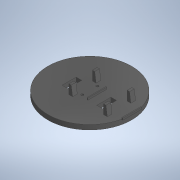
# Autodesk Inventor part: Swivel Top Drafting
Saved by Autodesk Inventor 2020.5 (Build 245400000, 400)
## iProperties
Part Number: Swivel Top Drafting
Material: Generic
Document SubType Name: Modeling
Designer: Wes
Appearance: Default
Author: Wes
Autodesk Inventor part; units mm, degrees
ref_plane "YZ Plane" through (0, 0, 0) normal (1, 0, 0) x (0, 1, 0)
ref_plane "XZ Plane" through (0, 0, 0) normal (0, 1, 0) x (-1, 0, 0)
ref_plane "XY Plane" through (0, 0, 0) normal (0, 0, 1) x (1, 0, 0)
sketch "Sketch1" plane through (0, 0, 0) normal (0, 0, 1) x (1, 0, 0)
  line L0 (0, 0) -> (0, 120) construction
  line L1 (-22.9924, 0) -> (-22.9924, 62) construction
  circle A0 centre (0, 31) radius 89
  line L2 (-20, 119) -> (20, 119)
  line L3 (20, 119) -> (20, 121)
  line L4 (20, 121) -> (-20, 121)
  line L5 (-20, 121) -> (-20, 119)
  line L6 (-20, 119) -> (20, 121) construction
  line L7 (20, 119) -> (-20, 121) construction
  line L8 (3.5475, 119) -> (3.5475, 78) construction
  line L9 (3.5475, 78) -> (3.5475, 66) construction
  line L10 (-20, 72) -> (-10, 72) construction
  line L11 (20, 72) -> (29, 72) construction
  line L12 (20, 66) -> (-10, 66)
  line L13 (-10, 66) -> (-10, 78)
  line L14 (-10, 78) -> (20, 78)
  line L15 (20, 78) -> (20, 66)
  line L16 (-20, 45.1356) -> (20, 45.1356)
  line L17 (20, 47.1356) -> (-20, 47.1356)
  line L18 (20, -7.8644) -> (-10, -7.8644)
  line L19 (-10, -7.8644) -> (-10, 4.1356)
  line L20 (-10, 4.1356) -> (20, 4.1356)
  line L21 (20, 4.1356) -> (20, -7.8644)
  line L22 (-20, 45.1356) -> (-20, 47.1356)
  line L23 (20, 45.1356) -> (20, 47.1356)
  line L24 (0, 31) -> (-16, 31) construction
  line L25 (0, 31) -> (16, 31) construction
  circle A1 centre (16, 31) radius 1.15
  circle A2 centre (-16, 31) radius 1.15
  point P0 (13.3041, 119)
  point P1 (-13.3041, 119)
  dimension "d0" = 120
  dimension "d1" = 62
  dimension "d2" = 40
  dimension "d3" = 2
  dimension "d4" = 41
  dimension "d5" = 12
  dimension "d6" = 10
  dimension "d7" = 9
  dimension "d8" = 30
  dimension "d9" = 12
  dimension "d10" = 40
  dimension "d11" = 2
  dimension "d12" = 30
  dimension "d13" = 12
  dimension "d18" = 16
  dimension "d19" = 16
  dimension "d20" = 2.3
  dimension "d21" = 2.3
  constraints: 52 end point, 8 horizontal, 7 parallel, 5 vertical, 4 perpendicular, 2 centre point, 2 coincident, 2 midpoint, 2 point on line, 3 other
  measures "d0" distance of L0.start L0.end
  measures "d1" distance of L1.start L1.end
  measures "d2" distance of L4.end L3.end
  measures "d3" distance of L3.end L2.end
  measures "d4" distance of L8.start L8.end
  measures "d5" distance of L8.end L9.end
  measures "d6" distance of L10.start L10.end
  measures "d7" distance of L11.start L11.end
  measures "d8" distance of L13.end L14.end
  measures "d9" distance of L12.end L13.end
  measures "d10" distance of L17.end L17.start
  measures "d11" distance of L17.start L16.end
  measures "d12" distance of L19.end L20.end
  measures "d13" distance of L19.start L19.end
  measures "d18" distance of L24.start L24.end
  measures "d19" distance of L24.start L25.end
  measures "d20" diameter of A1
  measures "d21" diameter of A2
extrude "Extrusion1" add sketch "Sketch1" along normal mid plane 10 contours A0 L2 | L2 A0 | L22 L17 L23 L16
sketch "Sketch2" plane through (0, 0, 5) normal (0, 0, 1) x (1, 0, 0)
  line L0 (20, 121) -> (-20, 121) projected
  line L1 (-20, 121) -> (-20, 119) projected
  line L2 (-20, 119) -> (20, 119) projected
  line L3 (20, 119) -> (20, 121) projected
  line L4 (20, 45.1356) -> (-20, 45.1356) projected
  line L5 (-20, 45.1356) -> (-20, 47.1356) projected
  line L6 (-20, 47.1356) -> (20, 47.1356) projected
  line L7 (20, 47.1356) -> (20, 45.1356) projected
  point P0 (0, 0)
extrude "Extrusion2" add sketch "Sketch2" along normal blind 4
sketch "Sketch3" plane through (0, 0, 5) normal (0, 0, 1) x (1, 0, 0)
  circle A0 centre (-16, 31) radius 2.65
  circle A1 centre (16, 31) radius 2.65
  point P0 (0, 0)
  dimension "d22" = 5.3
  dimension "d23" = 5.3
  constraints: 2 centre point, 2 coincident
  measures "d22" diameter of A0
  measures "d23" diameter of A1
extrude "Extrusion3" cut sketch "Sketch3" against normal blind 2.2
sketch "Sketch4" plane through (0, 31, -5) normal (0, 0, -1) x (-1, 0, 0)
  circle A0 centre (0, 0) radius 4
  point P0 (0, -31)
  dimension "d26" = 8
  constraints: 1 centre point
  measures "d26" diameter of A0
extrude "Extrusion4" cut sketch "Sketch4" against normal blind 1.1
sketch "Sketch5" plane through (0, 31, -5) normal (0, 0, -1) x (-1, 0, 0)
  circle A0 centre (0, 0) radius 5.975 construction
  circle A1 centre (0, 0) radius 7.5 construction
  arc A2 (4.225, 4.225) -> (-4.225, 4.225) centre (0, 0) ccw
  line L0 (-10.0244, 0) -> (9.4918, 0) construction
  arc A3 (-4.225, -4.225) -> (4.225, -4.225) centre (0, 0) ccw
  arc A4 (-5.3204, -5.2862) -> (5.3093, -5.2973) centre (0, 0) ccw
  line L1 (4.225, -4.225) -> (5.3093, -5.2973)
  line L2 (-4.225, -4.225) -> (-5.3204, -5.2862)
  arc A5 (5.3093, 5.2973) -> (-5.3204, 5.2862) centre (0, 0) ccw
  line L3 (4.225, 4.225) -> (5.3093, 5.2973)
  line L4 (-4.225, 4.225) -> (-5.3204, 5.2862)
  point P0 (0, -31)
  dimension "d30" = 15
  dimension "d29" = 11.95
  constraints: 10 end point, 10 point on circle, 5 centre point, 4 symmetric about line, 3 coincident, 1 concentric, 1 horizontal, 5 other
  measures "d29" diameter of A0
extrude "Extrusion5" add sketch "Sketch5" along normal blind 6.3
sketch "Sketch6" plane through (0, 31, -11.3) normal (0, 0, -1) x (-1, 0, 0)
  line L0 (0, 5.975) -> (0, 6.975) construction
  line L1 (0, 6.975) -> (0, 9.075) construction
  arc A0 (6.417, 6.417) -> (-6.417, 6.417) centre (0, 0) ccw
  arc A1 (4.9238, 4.9403) -> (-4.9321, 4.9321) centre (0, 0) ccw
  line L2 (-4.9321, 4.9321) -> (-6.417, 6.417)
  line L3 (4.9238, 4.9403) -> (6.417, 6.417)
  line L4 (-9.2245, 0) -> (9.451, 0) construction
  line L5 (0, -5.975) -> (0, -6.975) construction
  line L6 (0, -6.975) -> (0, -9.075) construction
  arc A2 (-6.417, -6.417) -> (6.417, -6.417) centre (0, 0) ccw
  arc A3 (-4.9321, -4.9321) -> (4.9238, -4.9403) centre (0, 0) ccw
  line L7 (-4.9321, -4.9321) -> (-6.417, -6.417)
  line L8 (4.9238, -4.9403) -> (6.417, -6.417)
  point P0 (0, -31)
  dimension "d34" = 1
  dimension "d36" = 2.1
  constraints: 18 end point, 10 point on circle, 9 symmetric about line, 4 centre point, 2 coincident, 2 vertical, 1 horizontal, 2 other
  measures "d34" distance of L0.end L0.start
  measures "d36" distance of L1.end L1.start
extrude "Extrusion6" add sketch "Sketch6" along normal blind 1.85
sketch "Sketch7" plane through (0, 31, -5) normal (0, 0, -1) x (-1, 0, 0)
  line L0 (-16, 0) -> (-16, 2.7) construction
  line L1 (-16, 0) -> (-16, -2.7) construction
  line L2 (-16, 0) -> (-10.25, 0) construction
  line L3 (-10.25, 0) -> (-10.25, 3.5) construction
  line L4 (-10.25, 0) -> (-10.25, -3.5) construction
  line L5 (-16, -2.7) -> (-10.25, -3.5)
  line L6 (-16, 2.7) -> (-10.25, 3.5)
  line L7 (-10.25, 3.5) -> (-10.5256, 5.4809)
  line L8 (-10.5256, 5.4809) -> (-16.2491, 4.4905)
  line L9 (-16.2491, 4.4905) -> (-16, 2.7)
  line L10 (-16, -2.7) -> (-16.2491, -4.6844)
  line L11 (-16.2491, -4.6844) -> (-10.5257, -5.4809)
  line L12 (-10.5257, -5.4809) -> (-10.25, -3.5)
  line L13 (0, -12.7277) -> (0, 17.2323) construction
  line L14 (16, 0) -> (16, 2.7) construction
  line L15 (16, 0) -> (16, -2.7) construction
  line L16 (16, 0) -> (10.25, 0) construction
  line L17 (10.25, 0) -> (10.25, 3.5) construction
  line L18 (10.25, 0) -> (10.25, -3.5) construction
  line L19 (16, -2.7) -> (10.25, -3.5)
  line L20 (16, 2.7) -> (10.25, 3.5)
  line L21 (10.25, 3.5) -> (10.5256, 5.4809)
  line L22 (10.5256, 5.4809) -> (16.2491, 4.4905)
  line L23 (16.2491, 4.4905) -> (16, 2.7)
  line L24 (16, -2.7) -> (16.2491, -4.6844)
  line L25 (16.2491, -4.6844) -> (10.5257, -5.4809)
  line L26 (10.5257, -5.4809) -> (10.25, -3.5)
  point P0 (0, -31)
  dimension "d41" = 2.7
  dimension "d42" = 2.7
  dimension "d43" = 5.75
  dimension "d44" = 3.5
  dimension "d45" = 3.5
  dimension "d46" = 2
  dimension "d47" = 2
  constraints: 54 end point, 11 symmetric about line, 5 vertical, 2 perpendicular, 1 horizontal
  measures "d41" distance of L0.start L0.end
  measures "d42" distance of L0.start L1.end
  measures "d43" distance of L2.start L2.end
  measures "d44" distance of L2.end L3.end
  measures "d45" distance of L2.end L4.end
  measures "d46" distance of L3.end L7.end
  measures "d47" distance of L1.end L10.end
extrude "Extrusion7" add sketch "Sketch7" along normal blind 2
fillet "Fillet1" [suppressed]
sketch "Sketch8" plane through (0, 0, 5) normal (0, 0, 1) x (1, 0, 0)
  line L0 (20, 45.1356) -> (-20, 45.1356) construction
  line L1 (-20, 45.1356) -> (-20, 16.6356) construction
  line L2 (-20, 16.6356) -> (-30, 16.6356)
  line L3 (-30, 16.6356) -> (-30, 21.6356)
  line L4 (-30, 21.6356) -> (-20, 21.6356)
  line L5 (-20, 16.6356) -> (-20, 21.6356)
  line L6 (-20, 119) -> (-20, 90.5) construction
  line L7 (-20, 90.5) -> (-30, 90.5)
  line L8 (-30, 90.5) -> (-30, 95.5)
  line L9 (-30, 95.5) -> (-20, 95.5)
  line L10 (-20, 90.5) -> (-20, 95.5)
  line L11 (0, -17.6167) -> (0, 154.2369) construction
  line L12 (20, 45.1356) -> (20, 16.6356) construction
  line L13 (20, 16.6356) -> (30, 16.6356)
  line L14 (30, 16.6356) -> (30, 21.6356)
  line L15 (30, 21.6356) -> (20, 21.6356)
  line L16 (20, 16.6356) -> (20, 21.6356)
  line L17 (20, 119) -> (20, 90.5) construction
  line L18 (20, 90.5) -> (30, 90.5)
  line L19 (30, 90.5) -> (30, 95.5)
  line L20 (30, 95.5) -> (20, 95.5)
  line L21 (20, 90.5) -> (20, 95.5)
  point P0 (0, 0)
  dimension "d50" = 28.5
  dimension "d51" = 10
  dimension "d52" = 5
  dimension "d53" = 28.5
  dimension "d54" = 10
  dimension "d55" = 5
  constraints: 42 end point, 9 symmetric about line, 5 vertical, 4 point on line, 2 collinear, 2 horizontal, 2 perpendicular
  measures "d50" distance of L0.end L1.end
  measures "d51" distance of L1.end L2.end
  measures "d52" distance of L2.end L3.end
  measures "d53" distance of L6.start L6.end
  measures "d54" distance of L6.end L7.end
  measures "d55" distance of L7.end L8.end
extrude "Extrusion8" add sketch "Sketch8" along normal blind 20
draft "FaceDraft1" angle 8 pull direction (0, 0, 1) faces at (-23.3333, 21.6356, 11.6667) (-23.3333, 95.5, 11.6667) (26.6667, 95.5, 11.6667) (26.6667, 21.6356, 11.6667) fixed edges at (-25, 21.6356, 25) (-25, 95.5, 25) (25, 95.5, 25) (25, 21.6356, 25)
body "Solid1"
